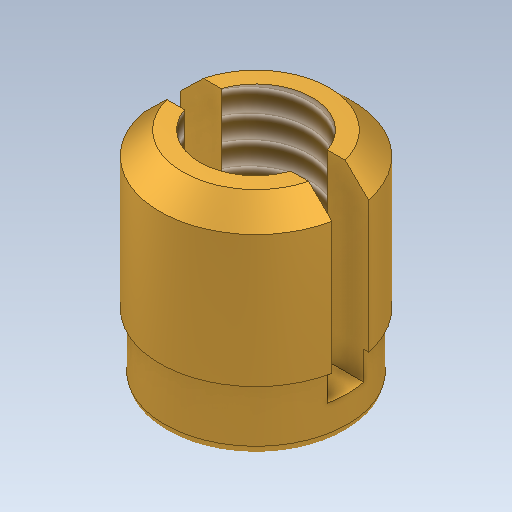
# Autodesk Inventor part: RS 278-534 M3 fixing Dia4FixHole
Saved by Autodesk Inventor 2021 (Build 250183000, 183)
## iProperties
Created: 2020-04-03
Part Number: RS 278-534 M3 fixing Dia4FixHole
Material: Brass, Soft Yellow
Document SubType Name: Modeling
Designer: jgray
Density: 8.47 g/cm^3
Appearance: Brass - Satin
Author: jgray
Autodesk Inventor part; units mm, degrees
ref_plane "YZ Plane" through (0, 0, 0) normal (1, 0, 0) x (0, 1, 0)
ref_plane "XZ Plane" through (0, 0, 0) normal (0, 1, 0) x (-1, 0, 0)
ref_plane "XY Plane" through (0, 0, 0) normal (0, 0, 1) x (1, 0, 0)
sketch "Sketch1" plane through (0, 0, 0) normal (0, 1, 0) x (-1, 0, 0)
  circle A0 centre (0, 0) radius 2.1
  dimension "d0" = 4.2
  constraints: 2 coincident, 1 centre point
  measures "d0" diameter of A0
extrude "Extrusion1" add sketch "Sketch1" along normal blind 4.78
hole "Hole1" at (0, 0, 0) direction (0, 1, 0) diameter 2.459 end through all thread size "M3x0.5" class "6H" standard "ISO Metric profile"
chamfer "Chamfer1" distance 0.5 angle 45 1 edges at (2.1, 4.78, 0)
sketch "Sketch2" plane through (0, 4.78, 0) normal (0, 1, 0) x (1, 0, 0)
  line L0 (2.1, -0.4) -> (-2.1, -0.4)
  line L1 (-2.1, -0.4) -> (-2.1, 0.4)
  line L2 (-2.1, 0.4) -> (2.1, 0.4)
  line L3 (2.1, 0.4) -> (2.1, -0.4)
  circle A0 centre (0, 0) radius 1.2295 projected
  line L4 (2.1, -0.4) -> (-2.1, 0.4) construction
  line L5 (-2.1, -0.4) -> (2.1, 0.4) construction
  circle A1 centre (0, 0) radius 2.1 projected
  point P0 (-2.1, 0)
  dimension "d13" = 0.8
  constraints: 12 end point, 3 midpoint, 2 parallel, 1 horizontal, 1 horizontal alignment, 1 perpendicular, 1 other
  measures "d13" distance of L0.end L1.end
extrude "Extrusion2" cut sketch "Sketch2" against normal blind 4 contours L0 A1 L3 | L0 A0 L2 A1 | A1 L2 L3 | L0 A0 L2 | A1 L2 A0 L0 | L0 L1 A1 | L1 L2 A1
sketch "Sketch3" plane through (0, 0, 0) normal (0, -1, 0) x (1, 0, 0)
  circle A0 centre (0, 0) radius 1.2295 projected
  line L0 (2.0616, 0.4) -> (1.1626, 0.4) projected
  circle A1 centre (0, 0) radius 2.1
  circle A2 centre (0, 0) radius 2
  dimension "d16" = 4
  constraints: 2 coincident, 1 centre point, 4 other
  measures "d16" diameter of A2
extrude "Extrusion3" cut sketch "Sketch3" against normal blind 1.4
fillet "Fillet1" radius 0.2 1 edges at (-2, 0, 0)
chamfer "Chamfer2" distance 0.3 angle 45 1 edges at (0, 0, 1.2295)
body "Solid1"
